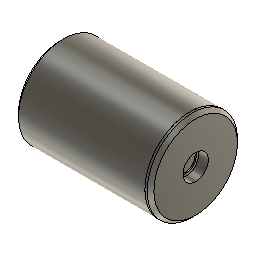
Rotor (Autodesk Fusion 360 design; units mm, degrees)
Autodesk Fusion 360 part; units mm, degrees
note: some values were not read from the file. Set by a fixed rule: which face or edge a step refers to.
sketch "Sketch1" plane through (0, 0, 0) normal (1, 0, 0) x (0, 1, 0)
  circle A0 centre (0, 0) radius 40
  dimension "d1" = 80
  constraint coincident A0.centre origin
  measures "d1" diameter of A0
extrude "Extrude1" add sketch "Sketch1" along normal blind 115 makes body 1
shell "Shell1" thickness 2 removed faces 1 at (115, 9.4847, -14.2223) on bodies 1
extrude "Extrude5" add 1 faces at (2, 0.6961, 10.9697) along direction (1, 0, 0) blind 8 on bodies 1 bodies 1
sketch "Sketch2" plane through (115, 0, 0) normal (1, 0, 0) x (0, 1, 0)
  circle A0 centre (0, 0) radius 38
  circle A1 centre (0, 0) radius 40
  circle A2 centre (0, 0) radius 37.7
  dimension "d8" = -0.3
extrude "Extrude3" add sketch "Sketch2" against normal blind 5 separate body contours A2 makes body 2
extrude "Extrude4" add sketch "Sketch2" along normal blind 5 contours A0 | A1 | A2 bodies 2
chamfer "Chamfer1" distance 3 angle 45 2 edges at (0, -37.2931, -14.4646) (120, -37.2931, -14.4646) on bodies 1 2
hole "Hole2" at (0, 0, 0) direction (1, 0, 0) diameter 22.4 depth 8.5 tip angle 180 bodies 1
hole "Hole1" at (120, 0, 0) direction (-1, 0, 0) diameter 22.4 depth 8.5 tip angle 180 bodies 2
hole "Hole3" at (8.5, 0, 0) direction (1, 0, 0) diameter 18 depth 1 tip angle 180 bodies 1
hole "Hole4" at (111.5, 0, 0) direction (-1, 0, 0) diameter 18 depth 1 tip angle 180 bodies 2
extrude "Extrude7" add 1 faces at (111.5, 1.0036, -10.3915) along direction (-1, 0, 0) blind 3 on bodies 2 bodies 2
extrude "Extrude8" add 1 faces at (110, 1.952, -0.1463) along direction (-1, 0, 0) up to surface (1.5 mm away) on bodies 2 bodies 2
chamfer "Chamfer2" distance 1.5 angle 45 1 edges at (110, -10.4421, -4.0501) on bodies 2
extrude "Extrude9" add 1 faces at (8.5, 1.0036, 10.3915) along direction (1, 0, 0) blind 3 on bodies 1 bodies 1
extrude "Extrude10" add 1 faces at (10, 0.3935, -4.2758) along direction (1, 0, 0) up to surface (1.5 mm away) on bodies 1 bodies 1
chamfer "Chamfer3" distance 1.5 angle 45 1 edges at (10, 10.4421, -4.0501) on bodies 1
